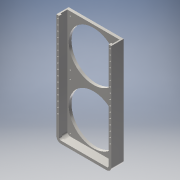
# Autodesk Inventor part: Cup_Dispenser_Hull
Saved by Autodesk Inventor 2016 (Build 200138000, 138)
## iProperties
Created: 2015-07-09
Part Number: Cup_Dispenser_Hull
Material: Generic
Document SubType Name: Modeling
Designer: marku
Density: 1 g/cm^3
Appearance: Titanium
Author: marku
Autodesk Inventor part; units mm, degrees
ref_plane "YZ Plane" through (0, 0, 0) normal (1, 0, 0) x (0, 1, 0)
ref_plane "XZ Plane" through (0, 0, 0) normal (0, 1, 0) x (-1, 0, 0)
ref_plane "XY Plane" through (0, 0, 0) normal (0, 0, 1) x (1, 0, 0)
sketch "Sketch1" plane through (0, 0, 0) normal (0, 1, 0) x (-1, 0, 0)
  line L0 (-60, 120) -> (60, 120)
  line L1 (60, 120) -> (60, -110)
  line L2 (50, -120) -> (-50, -120)
  line L3 (-60, -110) -> (-60, 120)
  line L4 (-60, 120) -> (60, -120) construction
  line L5 (60, 120) -> (-60, -120) construction
  line L6 (-60, 120) -> (60, 120)
  line L7 (60, 120) -> (60, 0)
  line L8 (60, 0) -> (-60, 0)
  line L9 (-60, 0) -> (-60, 120)
  line L10 (60, 0) -> (-60, 120) construction
  line L11 (-60, 0) -> (60, 120) construction
  circle A0 centre (0, 60) radius 54
  line L12 (54, 60) -> (60, 60) construction
  arc A1 (50, -120) -> (60, -110) centre (50, -110) ccw
  arc A2 (-60, -110) -> (-50, -120) centre (-50, -110) ccw
  point P0 (0, 0)
  dimension "d0" = 120
  dimension "d1" = 240
  dimension "d2" = 120
  dimension "d3" = 6
  dimension "d4" = 10
  constraints: 26 end point, 5 point on line, 4 midpoint, 4 parallel, 4 point on circle, 4 tangent, 3 horizontal, 2 centre point, 2 perpendicular, 1 equal radius, 1 horizontal alignment, 2 other
  measures "d0" distance of L4.end L5.end
  measures "d1" distance of L0.end L4.end
  measures "d2" distance between parallel lines of L8 L0
  measures "d3" distance of L12.start L12.end
  measures "d4" radius of A1
extrude "Extrusion1" add sketch "Sketch1" along normal blind 6
sketch "Sketch2" plane through (0, 0, 0) normal (0, -1, 0) x (1, 0, 0)
  circle A0 centre (0, 60) radius 54 construction
  line L0 (60, 120) -> (60, -110) projected
  line L1 (-60, 120) -> (60, 120) projected
  line L2 (-60, -110) -> (-60, 120) projected
  arc A1 (-60, -110) -> (-50, -120) centre (-50, -110) ccw projected
  line L3 (50, -120) -> (-50, -120) projected
  arc A2 (50, -120) -> (60, -110) centre (50, -110) ccw projected
  line L4 (57, -110) -> (57, 117)
  line L5 (57, 117) -> (-57, 117)
  line L6 (-57, 117) -> (-57, -110)
  arc A3 (-57, -110) -> (-50, -117) centre (-50, -110) ccw
  line L7 (-50, -117) -> (50, -117)
  arc A4 (50, -117) -> (57, -110) centre (50, -110) ccw
  line L8 (57, 117) -> (57, 120)
  line L9 (-57, 117) -> (-57, 120)
  point P0 (0, 0)
  dimension "d7" = 3
  constraints: 12 end point, 4 point on circle, 2 centre point, 2 point on line, 1 perpendicular, 1 vertical, 5 other
  measures "d7" distance between parallel lines of L0 L4
extrude "Extrusion2" add sketch "Sketch2" along normal blind 15 contours L0 A2 L3 A1 L2 L1 L9 L6 A3 L7 A4 L4 L8
sketch "Sketch3" plane through (0, -15, 0) normal (0, -1, 0) x (1, 0, 0)
  line L0 (60, -110) -> (60, 120) projected
  line L1 (60, 120) -> (57, 120) projected
  line L2 (57, 120) -> (57, -110) projected
  arc A0 (50, -117) -> (57, -110) centre (50, -110) ccw projected
  line L3 (50, -117) -> (-50, -117) projected
  arc A1 (-57, -110) -> (-50, -117) centre (-50, -110) ccw projected
  line L4 (-57, -110) -> (-57, 120) projected
  line L5 (-57, 120) -> (-60, 120) projected
  line L6 (-60, 120) -> (-60, -110) projected
  arc A2 (-60, -110) -> (-50, -120) centre (-50, -110) ccw projected
  line L7 (-50, -120) -> (50, -120) projected
  arc A3 (50, -120) -> (60, -110) centre (50, -110) ccw projected
  line L8 (57, 120) -> (54, 120)
  line L9 (-60, 120) -> (60, 120) construction
  line L10 (54, 120) -> (54, -110)
  line L11 (50, -114) -> (25, -114)
  arc A4 (50, -114) -> (54, -110) centre (50, -110) ccw
  line L12 (0, 0) -> (0, -136) construction
  line L13 (-57, 120) -> (-54, 120)
  line L14 (-54, 120) -> (-54, -110)
  line L15 (-50, -114) -> (25, -114)
  arc A5 (-54, -110) -> (-50, -114) centre (-50, -110) ccw
  dimension "d10" = 3
  constraints: 14 end point, 4 point on circle, 4 symmetric about line, 2 centre point, 2 parallel, 2 tangent, 1 coincident, 1 point on line, 1 vertical, 1 other
  measures "d10" distance between parallel lines of L2 L10
extrude "Extrusion3" add sketch "Sketch3" along normal blind 6
sketch "Sketch5" plane through (0, 6, 0) normal (0, 1, 0) x (1, 0, 0)
  circle A0 centre (0, -60) radius 54 projected
  line L0 (60, -120) -> (60, 110) projected
  arc A1 (60, 110) -> (50, 120) centre (50, 110) ccw projected
  line L1 (50, 120) -> (-50, 120) projected
  arc A2 (-50, 120) -> (-60, 110) centre (-50, 110) ccw projected
  line L2 (-60, 110) -> (-60, -120) projected
  line L3 (-60, -120) -> (60, -120) projected
  line L4 (-67.6504, 0) -> (67.3496, 0) construction
  circle A3 centre (0, 60) radius 54
  point P0 (0, 0)
  constraints: 2 end point, 1 centre point, 1 horizontal, 1 point on line, 1 symmetric about line, 1 other
extrude "Extrusion4" cut sketch "Sketch5" against normal up to next contours A3
sketch "Sketch6" plane through (0, 6, 0) normal (0, 1, 0) x (1, 0, 0)
  circle A0 centre (0, -60) radius 54 projected
  circle A1 centre (0, 60) radius 54 projected
  circle A2 centre (0, 60) radius 54 projected
  circle A3 centre (0, -60) radius 54 projected
  line L0 (60, -120) -> (60, 110) projected
  arc A4 (60, 110) -> (50, 120) centre (50, 110) ccw projected
  line L1 (50, 120) -> (-50, 120) projected
  arc A5 (-50, 120) -> (-60, 110) centre (-50, 110) ccw projected
  line L2 (-60, 110) -> (-60, -120) projected
  line L3 (-60, -120) -> (60, -120) projected
  line L4 (-50.0326, 0) -> (43.9674, 0) construction
  line L5 (0, -60) -> (-70, -60) construction
  line L6 (0, -60) -> (0, -118) construction
  point P0 (0, 0)
  point P1 (-51, -9)
  point P2 (-51, -111)
  point P3 (51, -9)
  point P4 (51, -111)
  point P5 (-51, 9)
  point P6 (-51, 111)
  point P7 (51, 111)
  point P8 (51, 9)
  dimension "d15" = 18
  dimension "d16" = 9
  constraints: 7 symmetric about line, 6 end point, 2 horizontal, 1 point on line, 1 vertical
  measures "d15" diameter of point (-51, -9) L4
  measures "d16" distance from line of L2 point (-51, -9)
hole "Hole1" at (-51, 6, 9) at (-51, 6, 111) at (51, 6, 111) at (51, 6, 9) at (-51, 6, -111) at (-51, 6, -9) at (51, 6, -111) at (51, 6, -9) direction (0, -1, 0) diameter 3.1 end through all
sketch "Sketch7" plane through (0, -21, 0) normal (0, -1, 0) x (1, 0, 0)
  line L0 (57, 120) -> (57, -110) construction
  line L1 (57, -110) -> (57, 120) projected
  line L2 (-57, -110) -> (-57, 120) construction
  line L3 (-57, 120) -> (-57, -110) projected
  line L4 (57, 120) -> (57, -110) projected
  line L5 (0, 119) -> (0, 0) construction
  point P0 (57, 60)
  point P1 (57, -60)
  point P2 (57, 114)
  point P3 (-57, 114)
  point P4 (-57, 102)
  point P5 (57, 102)
  point P6 (-57, 90)
  point P7 (57, 90)
  point P8 (-57, 78)
  point P9 (57, 78)
  point P10 (-57, 66)
  point P11 (57, 66)
  point P12 (-57, 54)
  point P13 (57, 54)
  point P14 (-57, 42)
  point P15 (57, 42)
  point P16 (-57, 30)
  point P17 (57, 30)
  point P18 (-57, 18)
  point P19 (57, 18)
  point P20 (-57, 6)
  point P21 (57, 6)
  point P22 (-57, -6)
  point P23 (57, -6)
  point P24 (-57, -18)
  point P25 (57, -18)
  point P26 (-57, -30)
  point P27 (57, -30)
  point P28 (-57, -42)
  point P29 (57, -42)
  point P30 (-57, -54)
  point P31 (57, -54)
  point P32 (-57, -66)
  point P33 (57, -66)
  dimension "d24" = 6
  dimension "d27" = 12
  constraints: 2 end point, 2 vertical, 1 point on line, 1 symmetric about line, 30 other
  measures "d24" distance of L0.start point (57, 114)
  measures "d27" distance of point (-57, 114) point (-57, 102)
hole "Hole2" at (57, -21, 114) at (-57, -21, 114) at (-57, -21, 102) at (57, -21, 102) at (-57, -21, 90) at (57, -21, 90) at (-57, -21, 78) at (57, -21, 78) at (-57, -21, 66) at (57, -21, 66) at (-57, -21, 54) at (57, -21, 54) at (-57, -21, 42) at (57, -21, 42) at (-57, -21, 30) at (57, -21, 30) at (-57, -21, 18) at (57, -21, 18) at (-57, -21, 6) at (57, -21, 6) at (-57, -21, -6) at (57, -21, -6) at (-57, -21, -18) at (57, -21, -18) at (-57, -21, -30) at (57, -21, -30) at (-57, -21, -42) at (57, -21, -42) at (-57, -21, -54) at (57, -21, -54) at (-57, -21, -66) at (57, -21, -66) direction (0, 1, 0) diameter 3.1 depth 4 tip angle 118
equation "\"d0\" = hull_width"
equation "\"d1\" = hull_length"
equation "\"d2\" = hull_width"
equation "\"d3\" = 2 * thickness"
equation "\"d4\" = roundness"
equation "\"d5\" = 2 * thickness"
equation "\"d7\" = thickness"
equation "\"d8\" = 5 * thickness"
equation "\"d10\" = thickness"
equation "\"d11\" = 2 * thickness"
equation "\"d13\" = 2 * thickness"
equation "\"d15\" = 6 * thickness"
equation "\"d16\" = 3 * thickness"
equation "\"d22\" = 1.33333 * thickness"
equation "\"d24\" = 2 * thickness"
equation "\"d27\" = 4 * thickness"
equation "\"d37\" = 1.33333 * thickness"
equation "\"thickness\" = 3"
equation "\"roundness\" = 10"
equation "\"hull_width\" = 120"
equation "\"hull_length\" = 2 * hull_width"
body "Solid1"
